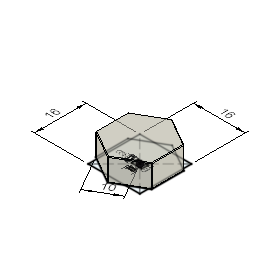
PolyButtonCap-v8 (Autodesk Fusion 360 design; units mm, degrees)
Autodesk Fusion 360 part; units mm, degrees
note: some values were not read from the file. Set by a fixed rule: which sketch regions a step uses; which face or edge a step refers to.
sketch "Sketch1" plane through (0, 0, 0) normal (0, 0, 1) x (1, 0, 0)
  line L0 (8, -8) -> (-8, -8)
  line L1 (-8, -8) -> (-8, 8)
  line L2 (-8, 8) -> (8, 8)
  line L3 (8, 8) -> (8, -8)
  line L4 (8, -8) -> (-8, 8) construction
  line L5 (-8, -8) -> (8, 8) construction
  line L6 (1.525, 1) -> (-1.525, 1)
  line L7 (-1.525, 1) -> (-1.525, -1)
  line L8 (-1.525, -1) -> (1.525, -1)
  line L9 (1.525, -1) -> (1.525, 1)
  line L10 (1.525, 1) -> (-1.525, -1) construction
  line L11 (-1.525, 1) -> (1.525, -1) construction
  line L12 (1.475, 1) -> (-1.475, 1)
  line L13 (-1.475, 1) -> (-1.475, -1)
  line L14 (-1.475, -1) -> (1.475, -1)
  line L15 (1.475, -1) -> (1.475, 1)
  line L16 (1.475, 1) -> (-1.475, -1) construction
  line L17 (-1.475, 1) -> (1.475, -1) construction
  line L18 (8.6603, -5) -> (8.6603, 5)
  line L19 (8.6603, 5) -> (0, 10)
  line L20 (0, 10) -> (-8.6603, 5)
  line L21 (-8.6603, 5) -> (-8.6603, -5)
  line L22 (-8.6603, -5) -> (0, -10)
  line L23 (0, -10) -> (8.6603, -5)
  dimension "d1" = 16
  dimension "d2" = 16
  dimension "d14" = 3.05
  dimension "d15" = 2
  dimension "d16" = 2.95
  dimension "d17" = 2
  dimension "d20" = 10
  constraint horizontal L0
  constraint perpendicular L0 L1
  constraint parallel L0 L2
  constraint parallel L1 L3
  constraint coincident L4 origin
  constraint coincident L5 origin
  constraint horizontal L6
  constraint perpendicular L6 L7
  constraint parallel L6 L8
  constraint parallel L7 L9
  constraint coincident L10 origin
  constraint coincident L11 origin
  constraint horizontal L12
  constraint perpendicular L12 L13
  constraint parallel L12 L14
  constraint parallel L13 L15
  constraint coincident L16 origin
  constraint coincident L17 origin
  constraint parallel L7 L21
  measures "d1" distance of L1.end L2.end
  measures "d2" distance of L0.end L1.end
  measures "d14" distance of L7.end L8.end
  measures "d15" distance of L6.end L7.end
  measures "d16" distance of L13.end L14.end
  measures "d17" distance of L12.end L13.end
  measures "d20" distance of origin L21.end
extrude "Extrude1" add sketch "Sketch1" along normal blind 7 contours L0 L22 L23 | L0 L1 L2 L3 L19 L20 L22 L23 | L3 L18 L19 L23 | L1 L20 L21 L22 | L2 L19 L20 | L6 L8 L9 L15 | L6 L8 L12 L13 L14 L15 | L6 L7 L8 L13
fillet "Fillet1" radius 0.2 7 faces at (-1.1547, -2.6667, 7) (1.1547, -9.3333, 2.3333) (8.6603, -1.6667, 4.6667) (-2.3094, -8.6667, 2.3333) (-8.6603, 1.6667, 4.6667) (-1.1547, 9.3333, 2.3333) (8.4402, 5.1271, 2.3333)
extrude "Extrude4" cut sketch "Sketch1" along normal blind 2.8 contours L6 L8 L9 L15 | L6 L8 L12 L13 L14 L15 | L6 L7 L8 L13
